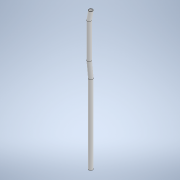
# Autodesk Inventor part: waterpipe
Saved by Autodesk Inventor 2020 (Build 240168000, 168)
## iProperties
Created: 2019-07-17
Part Number: waterpipe
Material: Generic
Document SubType Name: Modeling
Designer: ColinP
Density: 1 g/cm^3
Appearance: Default
Mass: 2.53385 g
Surface Area: 80.6132 cm^2
Volume: 2.53385 cm^3
Author: ColinP
Autodesk Inventor part; units mm, degrees
ref_plane "YZ Plane" through (0, 0, 0) normal (1, 0, 0) x (0, 1, 0)
ref_plane "XZ Plane" through (0, 0, 0) normal (0, 1, 0) x (-1, 0, 0)
ref_plane "XY Plane" through (0, 0, 0) normal (0, 0, 1) x (1, 0, 0)
sketch "Sketch1" plane through (0, 0, 0) normal (0, 1, 0) x (-1, 0, 0)
  circle A0 centre (0, 0) radius 3.175
  circle A1 centre (0, 0) radius 2.54
  dimension "d0" = 6.35
  dimension "d1" = 5.08
  constraints: 2 centre point, 2 coincident
  measures "d0" diameter of A0
  measures "d1" diameter of A1
extrude "Extrusion1" add sketch "Sketch1" along normal blind 127
sketch "Sketch7" plane through (0, 127, 0) normal (0, 1, 0) x (1, 0, 0)
  circle A0 centre (0, 0) radius 2.54 projected
  circle A1 centre (0, 0) radius 3.175 projected
sketch "Sketch15" plane through (0, 0, 0) normal (1, 0, 0) x (0, 1, 0)
  line L0 (153.67, 2.54) -> (209.55, 2.54)
  line L1 (222.25, 0) -> (209.55, 2.54)
  line L2 (153.67, 2.54) -> (127, 0)
  point P0 (0, 0)
  dimension "d48" = 55.88
  constraints: 6 end point
  measures "d48" distance of L0.start L0.end
sweep "Sweep8" add profiles "Sketch7" path "Sketch15" keep normal constant yes path curves L2 L0 L1
body "Solid1"
